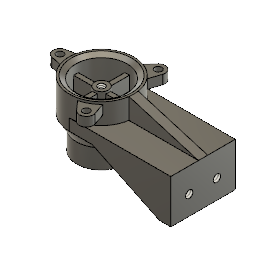
Task2g v0 (Autodesk Fusion 360 design; units mm, degrees)
Autodesk Fusion 360 part; units mm, degrees
sketch "Sketch1" plane through (0, 0, 0) normal (0, 1, 0) x (1, 0, 0)
  circle A0 centre (0, 0) radius 1.63
  circle A1 centre (0, 0) radius 1.38
  dimension "d1" = 3.26
  dimension "d2" = 2.76
  constraint coincident A0.centre A1.centre
  measures "d1" diameter of A0
  measures "d2" diameter of A1
extrude "Extrude1" add sketch "Sketch1" along normal blind 1.75 makes body 1
chamfer "Chamfer1" distance 0.25 angle 30 1 edges at (-1.2866, 1.75, -0.499) measured on face at (1.5355, 1.75, 0.1495) on bodies 1
sketch "Sketch2" plane through (0, 0, 0) normal (0, -1, 0) x (1, 0, 0)
  circle A0 centre (0, 0) radius 1.38
  circle A1 centre (0, 0) radius 1.63
  circle A2 centre (0, 0) radius 1.75
  dimension "d7" = 3.5
  constraint concentric A0 A2
  measures "d7" diameter of A2
extrude "Extrude2" add sketch "Sketch2" against normal blind 1.75 contours A2 bodies 1
sketch "Sketch3" plane through (0, 0, 0) normal (0, -1, 0) x (1, 0, 0)
  circle A0 centre (0, 0) radius 1.75
  circle A1 centre (0, 0) radius 1.38
  circle A2 centre (0, 0) radius 1.38
  circle A3 centre (0, 0) radius 1.75
  constraint coincident A0.centre A1.centre
  constraint concentric A0 A3
extrude "Extrude1'" add sketch "Sketch3" along normal blind 0.7 separate body makes body 2 in component "Component"
draft "Draft1" angle 30 neutral plane through (0, 0, 0) pull (0, 1, 0) 1 faces at (1.3731, -0.2333, -0.1374) on bodies 2 in component "Component"
draft "Draft2" angle -30 neutral plane through (0, 0, 0) pull (0, 1, 0) 1 faces at (1.7478, -0.4667, -0.0872) on bodies 2 in component "Component"
sketch "Sketch6" plane through (0, -0.7, 0) normal (0, -1, 0) x (1, 0, 0)
  circle A0 centre (0, 0) radius 0.9759
  circle A1 centre (0, 0) radius 1.3459
  circle A2 centre (0, 0) radius 1
  dimension "d16" = 2
  dimension "d19" = 1.9517
  constraint concentric A0 A2
  measures "d16" diameter of A2
  measures "d19" diameter of A0
extrude "Extrude2'" add sketch "Sketch6" along normal blind 1.05 contours A1 bodies 2 in component "Component"
sketch "Sketch7" plane through (0, 0, 0) normal (0, 1, 0) x (1, 0, 0)
  line L0 (1.39, 0.125) -> (-1.39, 0.125)
  line L1 (-1.39, 0.125) -> (-1.39, -0.125)
  line L2 (-1.39, -0.125) -> (1.39, -0.125)
  line L3 (1.39, -0.125) -> (1.39, 0.125)
  line L4 (1.39, 0.125) -> (-1.39, -0.125) construction
  line L5 (-1.39, 0.125) -> (1.39, -0.125) construction
  line L6 (0.125, -1.39) -> (0.125, 1.39)
  line L7 (-0.125, -1.39) -> (0.125, -1.39)
  line L8 (-0.125, 1.39) -> (-0.125, -1.39)
  line L9 (0.125, 1.39) -> (-0.125, 1.39)
  dimension "d20" = 2.78
  dimension "d21" = 0.25
  dimension "d22" = 2.78
  dimension "d23" = 0.25
  constraint perpendicular L0 L1
  constraint parallel L0 L2
  constraint parallel L1 L3
  constraint horizontal L0
  constraint coincident L4 origin
  constraint coincident L5 origin
  constraint perpendicular L6 L9
  constraint parallel L6 L8
  constraint parallel L7 L9
  measures "d20" distance of L1.end L2.end
  measures "d21" distance of L0.end L1.end
  measures "d22" distance of L8.start L7.start
  measures "d23" distance of L8.start L6.end
extrude "Extrude1''" add sketch "Sketch7" along normal blind 0.75 separate body makes body 3 in component "Component'"
move_body "Move1" bodies 3 to x (1, 0, 0) y (0, 1, 0) z (0, 0, 1) at (0, 0.375, 0) in component "Component'"
sketch "Sketch8" plane through (0, 1.125, 0) normal (0, 1, 0) x (-1, 0, 0)
  line L0 (-0.125, -1.39) -> (0.125, -1.39)
  line L1 (0.125, -1.39) -> (0.125, -0.125)
  line L2 (0.125, -0.125) -> (1.39, -0.125)
  line L3 (1.39, -0.125) -> (1.39, 0.125)
  line L4 (1.39, 0.125) -> (0.125, 0.125)
  line L5 (0.125, 0.125) -> (0.125, 1.39)
  line L6 (0.125, 1.39) -> (-0.125, 1.39)
  line L7 (-0.125, 1.39) -> (-0.125, 0.125)
  line L8 (-0.125, 0.125) -> (-1.39, 0.125)
  line L9 (-1.39, 0.125) -> (-1.39, -0.125)
  line L10 (-1.39, -0.125) -> (-0.125, -0.125)
  line L11 (-0.125, -0.125) -> (-0.125, -1.39)
  circle A0 centre (0, 0) radius 0.375
  constraint coincident A0.centre origin
extrude "Extrude2''" add sketch "Sketch8" along normal blind 0.125 and the other way blind 0.875 contours L10 L11 A0 | L1 L2 L4 L5 L7 L8 L10 L11 A0 | L1 L2 A0 | L7 L8 A0 | L4 L5 A0 bodies 3 in component "Component'"
sketch "Sketch10" plane through (0, 1.25, 0) normal (0, 1, 0) x (-1, 0, 0)
  circle A0 centre (0, 0) radius 0.375
  circle A1 centre (0, 0) radius 0.2188
  constraint concentric A0 A1
extrude "Extrude3" cut sketch "Sketch10" against normal through all contours A1 bodies 3 in component "Component'"
sketch "Sketch11" plane through (0, 1.75, 0) normal (0, 1, 0) x (-1, 0, 0)
  circle A0 centre (0, 0) radius 1.63
  circle A1 centre (0, 0) radius 1.75
  circle A2 centre (2.25, 0) radius 0.19
  circle A3 centre (2.25, 0) radius 0.375
  line L0 (1.6771, -0.5) -> (2.3252, -0.3674)
  line L1 (1.6771, 0.5) -> (2.3252, 0.3674)
  point P0 (1.75, 0)
  constraint coincident A1 L1.start
  constraint coincident A1 L0.start
  constraint concentric A2 A3
  constraint coincident A3 L0.end
  constraint tangent A3 L0
  constraint coincident A3 L1.end
  constraint tangent A3 L1
extrude "Extrude1'''" add sketch "Sketch11" against normal blind 0.625 separate body contours A1 A3 L0 L1 | A3 makes body 4 in component "Component''"
extrude "Extrude2'''" cut 1 faces at (-2.0659, 1.75, -0.2893) along direction (0, -1, 0) blind 0.125 on bodies 4 bodies 4 in component "Component''"
pattern_circular "C-Pattern1" count 3 over 360 about axis through (0, 1.25, 0) along (0, -1, 0) of "Extrude1'''", "Extrude2'''" makes body 5 at (1.2359, 1.4583, -2.1028) makes body 6 at (1.2031, 1.4583, 2.1217) in component "Component''"
sketch "Sketch12" plane through (0, 0, 0) normal (0, 1, 0) x (1, 0, 0)
  line L0 (0, 0) -> (0, 1.75)
  line L1 (0, 1.75) -> (5.5, 1.75)
  line L2 (5.5, 1.75) -> (5.5, -1.75)
  line L3 (5.5, -1.75) -> (0, -1.75)
  line L4 (0, -1.75) -> (0, 0)
  constraint coincident L0.start L4.end
  constraint vertical L0
  constraint perpendicular L0 L1
  constraint perpendicular L1 L2
  constraint perpendicular L2 L3
  constraint perpendicular L1 L4
extrude "Extrude3'" add sketch "Sketch12" along normal blind 0.63 separate body makes body 7
sketch "Sketch13" plane through (0, 0.63, 0) normal (0, 1, 0) x (-1, 0, 0)
  line L0 (0, 1.75) -> (-5.5, 1.75)
  line L1 (-5.5, 1.75) -> (-5.5, -1.75)
  line L2 (-5.5, -1.75) -> (0, -1.75)
  line L3 (0, -1.75) -> (0, 1.75)
  arc A0 (0, 1.75) -> (0, -1.75) centre (0, 0) ccw
  dimension "d52" = 3.5
  constraint coincident A0.centre origin
  measures "d52" diameter of A0
extrude "Extrude4" cut sketch "Sketch13" against normal through all contours L3 A0 bodies 7
sketch "Sketch14" plane through (0, 0.63, 0) normal (0, 1, 0) x (-1, 0, 0)
  arc A0 (0, 1.75) -> (0, -1.75) centre (0, 0) ccw
  line L0 (0, 1.75) -> (-5.5, 1.75)
  line L1 (-5.5, 1.75) -> (-5.5, -1.75)
  line L2 (-5.5, -1.75) -> (0, -1.75)
  line L3 (-5.5, 0) -> (-5.5, -0.25)
  line L4 (-5.5, -0.25) -> (-1.7, -0.25)
  line L5 (-1.7, -0.25) -> (-1.7, 0.25)
  line L6 (-1.7, 0.25) -> (-5.5, 0.25)
  line L7 (-5.5, -0.25) -> (-5.5, 0.25)
  constraint midpoint L1 L3.start
  constraint coincident L1 L3.end
  constraint perpendicular L1 L4
  constraint perpendicular L4 L5
  constraint coincident L1 L6.end
  constraint perpendicular L1 L6
extrude "Extrude5" add sketch "Sketch14" along normal blind 1.125 contours A0 L1 L3 L4 L6 L7 bodies 1 7
sketch "Sketch15" plane through (0, 0, 0.25) normal (0, 0, 1) x (1, 0, 0)
  line L0 (1.7321, 0.63) -> (5.5, 0.63)
  line L1 (5.5, 0.63) -> (5.5, 1.755)
  line L2 (5.5, 1.755) -> (1.7321, 1.755)
  line L3 (1.7321, 1.755) -> (1.7321, 1.75)
  line L4 (1.7321, 1.75) -> (1.7321, 0.63)
  line L5 (1.7321, 1.755) -> (5.5, 0.63)
  line L6 (5.5, 1.755) -> (1.7321, 1.755)
  line L7 (5.5, 1.755) -> (5.5, 0.63)
  constraint coincident L2.end L3.start
  constraint coincident L0.end L1.start
  constraint coincident L1.end L2.start
extrude "Extrude6" cut sketch "Sketch15" against normal through all contours L1 L2 L5 L6 L7 bodies 1
sketch "Sketch16" plane through (0, 0, 0) normal (0, -1, 0) x (1, 0, 0)
  arc A0 (0, 1.75) -> (0, -1.75) centre (0, 0) ccw
  line L0 (0, -1.75) -> (5.5, -1.75)
  line L1 (5.5, -1.75) -> (5.5, 1.75)
  line L2 (5.5, 1.75) -> (0, 1.75)
  circle A1 centre (0, 0) radius 1.38
  line L3 (5.5, 1.75) -> (1.25, 1.75)
  line L4 (1.25, 1.75) -> (1.25, -1.75)
  line L5 (1.25, -1.75) -> (5.5, -1.75)
  line L6 (5.5, 1.75) -> (5.5, -1.75)
  dimension "d60" = 4.25
  constraint coincident L1.end L2.start
  constraint perpendicular L1 L3
  constraint coincident L0 L4.end
  constraint perpendicular L0 L4
  constraint coincident L0.end L1.start
  measures "d60" distance of L1.end L3.end
extrude "Extrude7" add sketch "Sketch16" along normal blind 1.745 contours L0 L1 L2 A1 L3 L4 L5 L6 | A1 L4 picked at (1.2739, -0.1323) bodies 1
sketch "Sketch17" plane through (0, 0, 1.75) normal (0, 0, 1) x (1, 0, 0)
  line L0 (5.5, -1.745) -> (5.5, 0.63)
  line L1 (5.5, 0.63) -> (0, 0.63)
  line L2 (0, 0.63) -> (0, 0)
  line L3 (0, 0) -> (1.25, 0)
  line L4 (1.25, 0) -> (1.25, -1.745)
  line L5 (1.25, -1.745) -> (5.5, -1.745)
  line L6 (1.25, -1.745) -> (1.25, 0)
  line L7 (1.25, -1.745) -> (4.87, -1.745)
  line L8 (1.25, 0) -> (4.87, -1.745)
  dimension "d63" = 3.62
  constraint coincident L4.end L5.start
  constraint coincident L3.end L4.start
  constraint perpendicular L4 L7
  measures "d63" distance of L4.end L7.end
extrude "Extrude8" cut sketch "Sketch17" against normal through all contours L4 L5 L6 L7 L8 bodies 1
delete_face "DeleteFace1" 1 faces at (1.2739, 0, -0.1323) on bodies 1
sketch "Sketch18" plane through (5.5, 0, 0) normal (1, 0, 0) x (0, 0, -1)
  line L0 (0.25, 0.63) -> (-0.25, 0.63)
  line L1 (-0.25, 0.63) -> (-1.75, 0.63)
  line L2 (-1.75, 0.63) -> (-1.75, -1.745)
  line L3 (-1.75, -1.745) -> (1.75, -1.745)
  line L4 (1.75, -1.745) -> (1.75, 0.63)
  line L5 (1.75, 0.63) -> (0.25, 0.63)
  circle A0 centre (-0.75, -0.7) radius 0.25
  circle A1 centre (0.75, -0.7) radius 0.25
extrude "Extrude9" cut sketch "Sketch18" against normal blind 0.63 contours A0 | A1 bodies 1
thread "Thread1" "ANSI Unified Screw Threads 0.0177 45-254 UNM 2B" major diameter 0.4572 minor diameter 0.3683 pitch 0.1 angle 60 resizes the face on face at (-0.2177, 0.5833, -0.0218) on bodies 3 in component "Component'"
thread "Thread1'" "ANSI Unified Screw Threads 0.0197 50-203 UNM 2B" major diameter 0.508 minor diameter 0.3962 pitch 0.1251 angle 60 resizes the face on face at (5.08, -0.7125, -0.9997) on face at (5.08, -0.7125, 0.5003) on bodies 1
component "Component" placed x (1, 0, 0) y (0, 1, 0) z (0, 0, 1) at (0, 0, 0)
component "Component'" placed x (1, 0, 0) y (0, 1, 0) z (0, 0, 1) at (0, 0, 0)
component "Component''" placed x (1, 0, 0) y (0, 1, 0) z (0, 0, 1) at (0, 0, 0)
equation "d1 = ( 1.63 * 2 ) * 1 mm"
equation "d2 = ( 1.38 * 2 ) * 1 mm"
equation "d32 = 0.75 mm + 0.125 mm"
equation "d41 = -0.5 mm - 0.125 mm"
equation "d52 = 1.75 * 2 mm"
